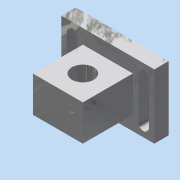
# Autodesk Inventor part: Stehlager 6mm
Saved by Autodesk Inventor 2015 (Build 190159000, 159)
## iProperties
Created: 2017-11-12
Part Number: Stehlager 6mm
Material: Generisch
Document SubType Name: Modeling
Designer: Christoph Soppa
Density: 1 g/cm^3
Appearance: Aluminium - dunkel
Author: Christoph Soppa
Autodesk Inventor part; units mm, degrees
ref_plane "YZ Plane" through (0, 0, 0) normal (1, 0, 0) x (0, 1, 0)
ref_plane "XZ Plane" through (0, 0, 0) normal (0, 1, 0) x (-1, 0, 0)
ref_plane "XY Plane" through (0, 0, 0) normal (0, 0, 1) x (1, 0, 0)
sketch "Skizze1" plane through (0, 0, 0) normal (0, 0, 1) x (1, 0, 0)
  line L0 (0, 0) -> (14, 0)
  line L1 (14, 0) -> (14, 14)
  line L2 (14, 14) -> (0, 14)
  line L3 (0, 14) -> (0, 0)
  circle A0 centre (7, 7) radius 3.05
  dimension "d0" = 14
  dimension "d1" = 14
  dimension "d2" = 6.1
  dimension "d3" = 7
  dimension "d4" = 7
  constraints: 8 end point, 2 parallel, 1 centre point, 1 horizontal, 1 perpendicular
  measures "d0" distance of L2.end L0.start
  measures "d1" distance of L1.end L2.end
  measures "d2" diameter of A0
  measures "d3" distance from line of L3 A0.centre
  measures "d4" distance from line of L0 A0.centre
extrude "Extrusion1" add sketch "Skizze1" along normal blind 10
sketch "Skizze2" plane through (0, 14, 0) normal (0, 1, 0) x (1, 0, 0)
  line L0 (-6, 4) -> (20, 4)
  line L1 (20, 4) -> (20, -14)
  line L2 (20, -14) -> (-6, -14)
  line L3 (-6, -14) -> (-6, 4)
  line L4 (14, 0) -> (0, 0) projected
  line L5 (0, 0) -> (0, -10) projected
  line L6 (14, -10) -> (0, -10) projected
  line L7 (14, 0) -> (14, -10) projected
  arc A0 (-1.5, 1) -> (-4.5, 1) centre (-3, 1) ccw
  arc A1 (-4.5, -11) -> (-1.5, -11) centre (-3, -11) ccw
  arc A2 (18.5, 1) -> (15.5, 1) centre (17, 1) ccw
  arc A3 (15.5, -11) -> (18.5, -11) centre (17, -11) ccw
  line L8 (-4.5, 1) -> (-4.5, -11)
  line L9 (-1.5, -11) -> (-1.5, 1)
  line L10 (15.5, -11) -> (15.5, 1)
  line L11 (18.5, -11) -> (18.5, 1)
  point P0 (0, 0)
  dimension "d7" = 6
  dimension "d8" = 6
  dimension "d9" = 4
  dimension "d10" = 4
  dimension "d11" = 3
  dimension "d12" = 3
  dimension "d13" = 3
  dimension "d14" = 3
  dimension "d15" = 3
  dimension "d16" = 3
  dimension "d17" = 3
  dimension "d18" = 3
  dimension "d19" = 3
  dimension "d20" = 3
  dimension "d21" = 3
  dimension "d22" = 3
  constraints: 16 end point, 8 point on circle, 8 tangent, 4 centre point, 2 parallel, 1 horizontal, 1 perpendicular
  measures "d7" distance between parallel lines of L3 L5
  measures "d8" distance between parallel lines of L7 L1
  measures "d9" distance between parallel lines of L0 L4
  measures "d10" distance between parallel lines of L6 L2
  measures "d11" diameter of A0
  measures "d12" diameter of A1
  measures "d13" diameter of A2
  measures "d14" diameter of A3
  measures "d15" distance from line of L0 A0.centre
  measures "d16" distance from line of L3 A0.centre
  measures "d17" distance from line of L3 A1.centre
  measures "d18" distance from line of L2 A1.centre
  measures "d19" distance from line of L2 A3.centre
  measures "d20" distance from line of L1 A3.centre
  measures "d21" distance from line of L1 A2.centre
  measures "d22" distance from line of L0 A2.centre
extrude "Extrusion2" add sketch "Skizze2" along normal blind 4 contours L0 L1 L2 L3 | L7 L6 L5 L4
